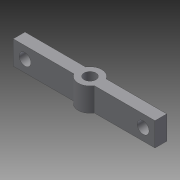
# Autodesk Inventor part: Y_Rail_Alignement _Connector_SquareBar-Rev3
Saved by Autodesk Inventor 2015 (Build 190159000, 159)
## iProperties
Created: 2017-01-11
Part Number: Y_Rail_Alignement _Connector_SquareBar-Rev3
Material: Generic
Document SubType Name: Modeling
Designer: Guy
Density: 1 g/cm^3
Appearance: Default
Author: Guy
Autodesk Inventor part; units mm, degrees
note: some values were not read from the file. Chosen so that the rebuilt part matches the saved one: sketch regions of "Extrusion1".
ref_plane "YZ Plane" through (0, 0, 0) normal (1, 0, 0) x (0, 1, 0)
ref_plane "XZ Plane" through (0, 0, 0) normal (0, 1, 0) x (-1, 0, 0)
ref_plane "XY Plane" through (0, 0, 0) normal (0, 0, 1) x (1, 0, 0)
sketch "Sketch1" plane through (0, 0, 0) normal (0, 0, 1) x (1, 0, 0)
  circle A0 centre (0, 0) radius 2.5
  circle A1 centre (0, 0) radius 5
  line L0 (-30, 2.5) -> (30, 2.5)
  line L1 (-30, -2.5) -> (30, -2.5)
  line L2 (30, -2.5) -> (30, 2.5)
  line L3 (-30, 2.5) -> (-30, -2.5)
  dimension "d0" = 5
  dimension "d1" = 10
  dimension "d2" = 5
  dimension "d3" = 2.5
  dimension "d4" = 60
  dimension "d5" = 30
  constraints: 8 end point, 2 centre point, 2 coincident, 2 horizontal, 1 parallel, 1 perpendicular
  measures "d0" diameter of A0
  measures "d1" diameter of A1
  measures "d2" distance between parallel lines of L1 L0
  measures "d3" distance from line of point (0, 0) L0
  measures "d4" distance between parallel lines of L3 L2
  measures "d5" distance from line of point (0, 0) L2
extrude "Extrusion1" add sketch "Sketch1" along normal blind 10 contours A0 L0 A1 L1 | A0 L1 A1 L0 | L0 A1 | L1 A1 | A1 L1 L3 L0 | L0 L2 L1 A1
sketch "Sketch2" plane through (4.3301, -2.5, 0) normal (0, -1, 0) x (1, 0, 0)
  line L0 (-8.6603, 10) -> (-8.6603, 0) projected
  line L1 (-34.3301, 10) -> (-8.6603, 10) projected
  line L2 (-34.3301, 0) -> (-34.3301, 10) projected
  line L3 (-8.6603, 0) -> (-34.3301, 0) projected
  line L4 (0, 0) -> (0, 10) projected
  line L5 (25.6699, 0) -> (0, 0) projected
  line L6 (25.6699, 0) -> (25.6699, 10) projected
  line L7 (0, 10) -> (25.6699, 10) projected
  circle A0 centre (-29.3301, 5) radius 2.5
  circle A1 centre (20.6699, 5) radius 2.5
  point P0 (-4.3301, 0)
  dimension "d8" = 5
  dimension "d9" = 5
  dimension "d10" = 5
  dimension "d11" = 5
  dimension "d12" = 5
  dimension "d13" = 5
  constraints: 2 centre point
  measures "d8" diameter of A1
  measures "d9" diameter of A0
  measures "d10" distance from line of L6 A1.centre
  measures "d11" distance from line of L2 A0.centre
  measures "d12" distance from line of L1 A0.centre
  measures "d13" distance from line of L7 A1.centre
extrude "Extrusion2" cut sketch "Sketch2" against normal blind 10 contours A0 | A1
body "Solid1"
